2e1efe84-0719-491b-89a8-e3191c542451 (Autodesk Fusion 360 design; units mm, degrees)
Autodesk Fusion 360 part; units mm, degrees
note: some values were not read from the file. Set by a fixed rule: which sketch regions a step uses.
sketch "Sketch1" plane through (0, 0, 0) normal (0, 1, 0) x (1, 0, 0)
  circle A0 centre (0, 0) radius 12.7
  circle A1 centre (0, 0) radius 13.97
  circle A2 centre (0, 0) radius 11.43
  circle A3 centre (0, 0) radius 11.9341
  arc A4 (13.9342, -0.9995) -> (-12.8046, -5.5861) centre (0, 0) ccw
  circle A5 centre (0, 0) radius 7.1437
  line L0 (0, 0) -> (13.97, 0) construction
  line L1 (0, 0) -> (-1.0401, -11.8887)
  line L2 (0, 0) -> (-2.0723, -11.7528)
  line L3 (0, 0) -> (-3.0888, -11.5275)
  line L4 (0, 0) -> (-4.0817, -11.2144)
  line L5 (0, 0) -> (-5.0436, -10.816)
  line L6 (0, 0) -> (-5.967, -10.3352)
  line L7 (0, 0) -> (-6.8451, -9.7758)
  line L8 (-1.0401, -11.8887) -> (-0.0026, -11.9795) construction
  line L9 (-2.0723, -11.7528) -> (-0.0211, -12.1145) construction
  line L10 (-3.0888, -11.5275) -> (-0.0709, -12.3361) construction
  line L11 (-4.0817, -11.2144) -> (-0.1671, -12.6392) construction
  line L12 (-5.0436, -10.816) -> (-0.3242, -13.0166) construction
  line L13 (-5.967, -10.3352) -> (-0.5555, -13.4596) construction
  line L14 (-6.8451, -9.7758) -> (-0.8734, -13.9573) construction
  line L15 (0, 0) -> (-7.6711, -9.142)
  line L16 (-7.6711, -9.142) -> (-1.2887, -14.4975) construction
  line L17 (0, 0) -> (-8.4387, -8.4387)
  line L18 (-8.4387, -8.4387) -> (-1.811, -15.0664) construction
  spline S0 degree 5 poles (-1.811, -15.0664) (-1.7952, -15.0465) (-1.7634, -15.007) (-1.715, -14.9493) (-1.6489, -14.875) (-1.5648, -14.7858) (-1.4804, -14.699) (-1.3969, -14.6134) (-1.3155, -14.5278) (-1.2374, -14.4412) (-1.1628, -14.3534) (-1.092, -14.2643) (-1.0245, -14.1742) (-0.9599, -14.0838) (-0.8977, -13.9935) (-0.8374, -13.9041) (-0.7788, -13.8157) (-0.7218, -13.7285) (-0.6667, -13.6424) (-0.6136, -13.5572) (-0.5628, -13.4728) (-0.5144, -13.3891) (-0.4686, -13.3061) (-0.4252, -13.2239) (-0.3842, -13.1428) (-0.3455, -13.0628) (-0.309, -12.9843) (-0.2746, -12.9074) (-0.2423, -12.8321) (-0.2122, -12.7585) (-0.1843, -12.6866) (-0.1586, -12.6165) (-0.1352, -12.5483) (-0.1138, -12.4825) (-0.0945, -12.4192) (-0.077, -12.3588) (-0.0613, -12.3013) (-0.0475, -12.2469) (-0.0357, -12.1954) (-0.0262, -12.1468) (-0.0188, -12.1015) (-0.0131, -12.0599) (-0.0087, -12.0234) (-0.0048, -11.993) (-0.0012, -11.9694) (0.0017, -11.9523) (0.0026, -11.943) (0.0019, -11.9379) (0.0007, -11.9352) (0, -11.9341) knots 0 0 0 0 0 0 0.022222 0.044444 0.066667 0.088889 0.111111 0.133333 0.155556 0.177778 0.2 0.222222 0.244444 0.266667 0.288889 0.311111 0.333333 0.355556 0.377778 0.4 0.422222 0.444444 0.466667 0.488889 0.511111 0.533333 0.555556 0.577778 0.6 0.622222 0.644444 0.666667 0.688889 0.711111 0.733333 0.755556 0.777778 0.8 0.822222 0.844444 0.866667 0.888889 0.911111 0.933333 0.955556 0.977778 1 1 1 1 1 1
  line L19 (-1.9071, -15.1882) -> (-1.7148, -14.9446)
  line L20 (0.0373, -11.9925) -> (-0.0373, -11.8757)
  line L21 (-0.1892, -12.6986) -> (0, 0)
  line L22 (0, 0) -> (-0.5753, -6.1386) construction
  line L23 (0, -11.9341) -> (0, 0) construction
  spline S1 degree 5 poles (0, -11.9341) (0, -11.8998) (0, -11.8374) (0, -11.7626) (0, -11.6937) (0, -11.6291) (0, -11.5695) (0, -11.508) (0, -11.4576) (0, -11.43) knots 0 0 0 0 0 0 0.2 0.4 0.6 0.8 1 1 1 1 1 1
  spline S2 degree 5 poles (-2.2173, -11.7263) (-2.2109, -11.6926) (-2.1993, -11.6313) (-2.1854, -11.5578) (-2.1726, -11.4901) (-2.1606, -11.4266) (-2.1495, -11.368) (-2.1381, -11.3077) (-2.1287, -11.2581) (-2.1236, -11.231) knots 0 0 0 0 0 0 0.2 0.4 0.6 0.8 1 1 1 1 1 1
  line L24 (0, -12.0221) -> (0, -11.8461)
  line L25 (0, -11.5007) -> (0, -11.3593)
  line L26 (-2.2336, -11.8128) -> (-2.2009, -11.6399)
  line L27 (-2.1367, -11.3005) -> (-2.1105, -11.1615)
  spline S3 degree 5 poles (-1.0198, -15.1405) (-1.0316, -15.118) (-1.0555, -15.0734) (-1.0923, -15.0077) (-1.1434, -14.9224) (-1.2095, -14.8191) (-1.2764, -14.7181) (-1.3425, -14.6185) (-1.4065, -14.5192) (-1.4673, -14.4197) (-1.5242, -14.3195) (-1.5772, -14.2188) (-1.6268, -14.1177) (-1.6735, -14.0169) (-1.7179, -13.9167) (-1.7605, -13.8176) (-1.8016, -13.7199) (-1.8414, -13.6236) (-1.8795, -13.5287) (-1.9159, -13.4352) (-1.9501, -13.3428) (-1.9821, -13.2516) (-2.0117, -13.1615) (-2.0391, -13.0727) (-2.0643, -12.9853) (-2.0875, -12.8996) (-2.1088, -12.8157) (-2.1283, -12.7337) (-2.1461, -12.6537) (-2.162, -12.5757) (-2.176, -12.4999) (-2.1882, -12.4263) (-2.1986, -12.355) (-2.2073, -12.2863) (-2.2146, -12.2205) (-2.2205, -12.1579) (-2.2253, -12.0985) (-2.2287, -12.0425) (-2.2307, -11.9897) (-2.2311, -11.9402) (-2.2299, -11.8942) (-2.2277, -11.8524) (-2.2253, -11.8157) (-2.2235, -11.7851) (-2.2227, -11.7612) (-2.2224, -11.7439) (-2.2215, -11.7346) (-2.2198, -11.7297) (-2.2182, -11.7273) (-2.2173, -11.7263) knots 0 0 0 0 0 0 0.022222 0.044444 0.066667 0.088889 0.111111 0.133333 0.155556 0.177778 0.2 0.222222 0.244444 0.266667 0.288889 0.311111 0.333333 0.355556 0.377778 0.4 0.422222 0.444444 0.466667 0.488889 0.511111 0.533333 0.555556 0.577778 0.6 0.622222 0.644444 0.666667 0.688889 0.711111 0.733333 0.755556 0.777778 0.8 0.822222 0.844444 0.866667 0.888889 0.911111 0.933333 0.955556 0.977778 1 1 1 1 1 1
  line L28 (-0.9479, -15.2781) -> (-1.0917, -15.003)
  line L29 (-2.2647, -11.7768) -> (-2.1698, -11.6758)
  point P0 (-0.1892, -12.6986)
  point P1 (0, -11.43)
  point P2 (-1.4272, -14.4845)
  point P3 (-1.735, -13.8765)
  point P4 (-1.9548, -13.3284)
  point P5 (-2.0998, -12.8502)
  point P6 (-2.184, -12.4502)
  point P7 (-2.2223, -12.1345)
  point P8 (-2.2301, -11.9075)
  point P9 (-2.2231, -11.7714)
  point P10 (-2.1236, -11.231)
  dimension "d2" = 27.94
  dimension "id" = 22.86
  dimension "BaseDiameter" = 23.8682
  dimension "d1" = 14.2875
  dimension "d34" = 5
  dimension "d35" = 5
  dimension "d36" = 5
  dimension "d37" = 5
  dimension "d38" = 5
  dimension "d39" = 5
  dimension "d41" = 1.0414
  dimension "d42" = 2.0829
  dimension "d43" = 3.1243
  dimension "d44" = 4.1658
  dimension "d45" = 5.2072
  dimension "d46" = 6.2487
  dimension "d47" = 7.2901
  dimension "d48" = 5
  dimension "d49" = 8.3316
  dimension "d50" = 5
  dimension "d51" = 9.373
  dimension "d55" = 4.5
  dimension "d60" = 5
  constraint coincident A0.centre A1.centre
  constraint concentric A0 A2
  constraint coincident A1 A4.end
  constraint horizontal L0
  constraint coincident A4 L0.end
  constraint coincident A3 S0.end
  constraint coincident A3 L1.end
  constraint coincident A3 L2.end
  constraint coincident A3 L3.end
  constraint coincident A3 L4.end
  constraint coincident A3 L5.end
  constraint coincident A3 L6.end
  constraint coincident A3 L7.end
  constraint vertical A0.centre S0.end
  constraint tangent A3 L8
  constraint tangent A3 L9
  constraint tangent A3 L10
  constraint tangent A3 L11
  constraint tangent A3 L12
  constraint tangent A3 L13
  constraint tangent A3 L14
  constraint coincident A3 L15.end
  constraint tangent A3 L16
  constraint coincident A3 L17.end
  constraint tangent A3 L18
  constraint midpoint L18.end L19
  constraint midpoint S0.end L20
  constraint coincident A0 P0
  constraint coincident S0 P0
  constraint coincident P0 L21.start
  constraint coincident L23 P1
  constraint coincident A2 P1
  constraint coincident P1 S1.end
  constraint midpoint S0.end L24
  constraint midpoint P1 L25
  constraint symmetric S0.end L22 S2.start
  constraint symmetric L8.end L22 P9
  constraint symmetric L9.end L22 P8
  constraint symmetric L10.end L22 P7
  constraint symmetric L11.end L22 P6
  constraint symmetric L12.end L22 P5
  constraint symmetric L13.end L22 P4
  constraint symmetric L14.end L22 P3
  constraint symmetric L16.end L22 P2
  constraint symmetric L18.end L22 S3.start
  constraint symmetric L19.start L22 L28.start
  constraint symmetric L19.end L22 L28.end
  constraint symmetric L20.start L22 L29.start
  constraint symmetric L20.end L22 L29.end
  constraint symmetric L22 P1 P10
  constraint symmetric L22 L24.start L26.start
  constraint symmetric L22 L24.end L26.end
  constraint symmetric L22 L25.start L27.start
  constraint symmetric L22 L25.end L27.end
  constraint vertical L24
  constraint vertical L25
  measures "d2" diameter of A1
  measures "id" diameter of A2
  measures "BaseDiameter" diameter of A3
  measures "d1" diameter of A5
  measures "d34" angle of L1 L2
  measures "d35" angle of L2 L3
  measures "d36" angle of L3 L4
  measures "d37" angle of L4 L5
  measures "d38" angle of L5 L6
  measures "d39" angle of L6 L7
  measures "d41" distance of L1.end L8.end
  measures "d42" distance of L2.end L9.end
  measures "d43" distance of L3.end L10.end
  measures "d44" distance of L4.end L11.end
  measures "d45" distance of L5.end L12.end
  measures "d46" distance of L6.end L13.end
  measures "d47" distance of L7.end L14.end
  measures "d48" angle of L7 L15
  measures "d49" distance of L15.end L16.end
  measures "d50" angle of L15 L17
  measures "d51" distance of L17.end L18.end
  measures "d55" angle of L21 L22
  measures "d60" angle of L1 L23
extrude "Extrude1" add sketch "Sketch1" along normal blind 304.8 contours A0 A1 S0 S3 | A3 S0 L21 L24 | A0 A3 L21 L26 S3 | A2 A3 L21 S1 L24 L25 | A2 A3 L1 L21 | A2 A3 L1 L2 | A2 A3 L2 S2 L26 L27 makes body 1
pattern_circular "C-Pattern2" count 12 over 360 about axis through (0, 1.75, 0) along (0, 1, 0) of bodies 1 makes body 2 at (5.5082, 203.2, 10.0152) makes body 3 at (9.7779, 203.2, 5.9193) makes body 4 at (11.3906, 203.2, 0.9483) makes body 5 at (10.3387, 203.2, -4.8741) makes body 6 at (5.9193, 203.2, -9.7779) makes body 7 at (0.9483, 203.2, -11.3906) makes body 8 at (-5.5082, 203.2, -10.0152) makes body 9 at (-9.3904, 203.2, -6.5165) makes body 10 at (-11.3906, 203.2, -0.9483) makes body 11 at (-10.0152, 203.2, 5.5082) makes body 12 at (-6.5165, 203.2, 9.3904)
extrude "Extrude2" add sketch "Sketch1" along normal blind 304.8 contours A2 A5 L17 L21 | A2 A5 L1 L21 | A2 A5 L1 L2 | A2 A5 L2 L3 | A2 A5 L3 L4 | A2 A5 L15 L17 | A2 A5 L4 L5 | A2 A5 L5 L6 | A2 A5 L6 L7 | A2 A5 L7 L15 bodies 1 2 3 4 5 6 7 8 9 10 11 12
ref_plane "WorkPlane1" through (6.2747, 152.4, -0.8261) normal (0.130526, 0, 0.991445) x (0.991445, 0, -0.130526)
fillet "Fillet1" [suppressed]
mirror "Mirror3" [suppressed]
pattern_circular "C-Pattern1" [suppressed]
equation "d = 1 in"
equation "OutsideDiameter = d2"
equation "PitchDiameter = d"
equation "id = PitchDiameter - 2 * ( PitchDiameter / TeethNumber )"
equation "BaseDiameter = PitchDiameter * cos(20 deg)"
equation "Length = 12 in"
equation "t = 20"
equation "ShaftDiameter = d1"
equation "TeethNumber = t"
equation "Pitch = 32"
equation "d30 = ( 1.25 * ( PitchDiameter / TeethNumber ) ) - ( PitchDiameter / TeethNumber )"
equation "Basecircum = PI * PitchDiameter * cos(20 deg)"
equation "d41 = Basecircum * 5 / 360"
equation "d42 = Basecircum * 10 / 360"
equation "d43 = Basecircum * 15 / 360"
equation "d44 = Basecircum * 20 / 360"
equation "d45 = Basecircum * 25 / 360"
equation "d46 = Basecircum * 30 / 360"
equation "d47 = Basecircum * 35 / 360"
equation "d49 = Basecircum * 40 / 360"
equation "d51 = Basecircum * 45 / 360"
equation "d55 = ( 360 / ( 4 * TeethNumber ) ) * 1 deg"
